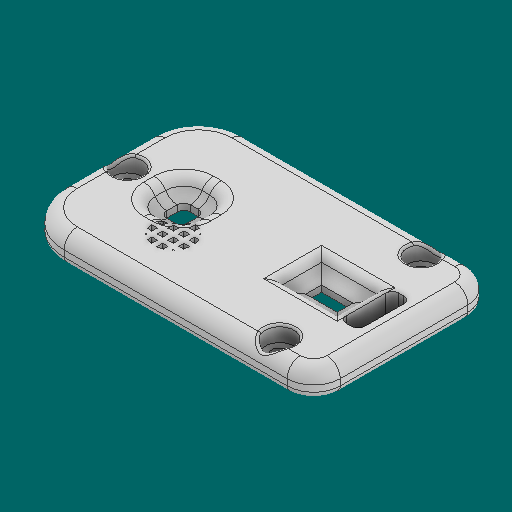
# Autodesk Inventor part: vape back
Saved by Autodesk Inventor 2025.1 (Build 291241000, 241)
## iProperties
Created: 2026-08-30
Part Number: vape back
Material: Generic
Document SubType Name: Modeling
Designer: Luke Buonanno
Density: 1 g/cm^3
Appearance: Default
Author: Luke Buonanno
Autodesk Inventor part; units mm, degrees
ref_plane "YZ Plane" through (0, 0, 0) normal (1, 0, 0) x (0, 1, 0)
ref_plane "XZ Plane" through (0, 0, 0) normal (0, 1, 0) x (-1, 0, 0)
ref_plane "XY Plane" through (0, 0, 0) normal (0, 0, 1) x (1, 0, 0)
sketch "Sketch1" plane through (0, 0, 0) normal (1, 0, 0) x (0, 1, 0)
  point P0 (0, 0)
sketch "Sketch2" plane through (0, 0, 0) normal (0, 1, 0) x (-1, 0, 0)
  point P0 (0, 0)
sketch "Sketch3" plane through (0, 0, 0) normal (0, 1, 0) x (-1, 0, 0)
  line L0 (24.5772, 9.7458) -> (-30.4138, 9.7458)
  line L1 (-30.4138, 9.7458) -> (-30.4138, -21.7502)
  line L2 (-30.4138, -21.7502) -> (24.5772, -21.7502)
  line L3 (24.5772, -21.7502) -> (24.5772, 9.7458)
  point P0 (0, 0)
  dimension "d0" = 54.991
  dimension "d1" = 31.496
  constraints: 8 end point, 2 parallel, 1 horizontal, 1 perpendicular
  measures "d0" distance of L1.end L2.end
  measures "d1" distance of L2.end L0.start
extrude "Extrusion1" add sketch "Sketch3" along normal blind 5
sketch "Sketch4" plane through (0, 5, 0) normal (0, 1, 0) x (1, 0, 0)
  line L0 (-24.5772, 21.7502) -> (-24.5772, -9.7458) projected
  line L1 (-24.5772, 6.0022) -> (-22.3166, 6.0022)
  circle A0 centre (-22.3166, 6.0022) radius 2.8
  point P0 (0, 0)
  dimension "d4" = 2.2606
  dimension "d5" = 5.6
  constraints: 2 end point, 1 centre point, 1 coincident, 1 horizontal, 1 midpoint
  measures "d4" distance of L1.start L1.end
  measures "d5" diameter of A0
sketch "Sketch5" plane through (0, 5, 0) normal (0, 1, 0) x (1, 0, 0)
  line L0 (30.4138, -9.7458) -> (30.4138, 21.7502) projected
  line L1 (30.4138, 21.7502) -> (-24.5772, 21.7502) projected
  line L2 (-24.5772, 21.7502) -> (-24.5772, -9.7458) projected
  line L3 (-24.5772, -9.7458) -> (30.4138, -9.7458) projected
  line L4 (30.4138, -11.2458) -> (-26.0772, -11.2458)
  line L5 (-26.0772, -11.2458) -> (-26.0772, 23.2502)
  line L6 (-26.0772, 23.2502) -> (30.4138, 23.2502)
  line L7 (30.4138, 23.2502) -> (30.4138, -11.2458)
  line L8 (30.4138, -11.2458) -> (-26.0772, 23.2502) construction
  line L9 (-26.0772, -11.2458) -> (30.4138, 23.2502) construction
  point P0 (0, 0)
  point P1 (2.1683, 6.0022)
  dimension "d6" = 1.5
  dimension "d7" = 1.5
  dimension "d8" = 1.5
  dimension "d9" = 0
  constraints: 12 end point, 2 midpoint, 2 parallel, 1 horizontal, 1 perpendicular
  measures "d6" distance between parallel lines of L5 L2
  measures "d7" distance between parallel lines of L6 L1
  measures "d8" distance between parallel lines of L4 L3
  measures "d9" distance between parallel lines of L0 L7
extrude "Extrusion2" add sketch "Sketch5" against normal blind 5
extrude "Extrusion3" cut sketch "Sketch4" against normal blind 3
sketch "Sketch6" plane through (-22.3166, 2, -6.0022) normal (0, 1, 0) x (1, 0, 0)
  circle A0 centre (0, 0) radius 2.8 projected
  circle A1 centre (0, 0) radius 1.5
  point P0 (22.3166, -6.0022)
  dimension "d14" = 3
  constraints: 1 centre point, 1 coincident
  measures "d14" diameter of A1
extrude "Extrusion4" cut sketch "Sketch6" against normal blind 3 contours A1
sketch "Sketch7" plane through (0, 5, 0) normal (0, 1, 0) x (1, 0, 0)
  circle A0 centre (-22.3166, 6.0022) radius 2.8 projected
  line L0 (30.4138, -11.2458) -> (30.4138, 23.2502) projected
  line L1 (30.4138, 23.2502) -> (-26.0772, 23.2502) projected
  line L2 (-26.0772, -11.2458) -> (30.4138, -11.2458) projected
  line L3 (30.4138, -9.7458) -> (-22.3166, -9.7458)
  line L4 (-22.3166, -9.7458) -> (-22.3166, 21.7502)
  line L5 (-22.3166, 21.7502) -> (30.4138, 21.7502)
  line L6 (30.4138, 21.7502) -> (30.4138, -9.7458)
  line L7 (30.4138, -9.7458) -> (-22.3166, 21.7502) construction
  line L8 (-22.3166, -9.7458) -> (30.4138, 21.7502) construction
  line L9 (30.4138, -9.7458) -> (9.8906, -9.7458)
  line L10 (20.1522, -9.7458) -> (20.1522, 21.7502)
  line L11 (20.1522, -9.7458) -> (20.1522, -7.4852)
  line L12 (20.1522, 21.7502) -> (20.1522, 19.4896)
  circle A1 centre (20.1522, -7.4852) radius 2.75
  circle A2 centre (20.1522, 19.4896) radius 2.75
  point P0 (0, 0)
  point P1 (4.0486, 6.0022)
  dimension "d17" = 1.5
  dimension "d18" = 1.5
  dimension "d19" = 0
  dimension "d20" = 10.2616
  dimension "d21" = 2.2606
  dimension "d22" = 2.2606
  dimension "d23" = 5.5
  dimension "d24" = 5.5
  dimension "d25" = 5.6
  constraints: 20 end point, 4 point on line, 3 midpoint, 2 centre point, 2 coincident, 2 parallel, 2 perpendicular, 1 horizontal
  measures "d17" distance between parallel lines of L1 L5
  measures "d18" distance between parallel lines of L2 L3
  measures "d19" distance between parallel lines of L0 L6
  measures "d20" distance of L3.start L10.start
  measures "d21" distance of L10.start L11.end
  measures "d22" distance of L10.end L12.end
  measures "d23" diameter of A1
  measures "d24" diameter of A2
  measures "d25" diameter of A0
extrude "Extrusion5" cut sketch "Sketch7" against normal blind 3 contours A2 L5 | L5 L10 A2 | L5 A2 L10 | A1 L10 L3 | L3 A1 | A1 L3 L10
sketch "Sketch8" plane through (20.1522, 2, 7.4852) normal (0, 1, 0) x (1, 0, 0)
  circle A0 centre (0, 0) radius 2.75 projected
  circle A1 centre (0, 0) radius 1.5
  circle A2 centre (0, 26.9748) radius 2.75 projected
  circle A3 centre (0, 26.9748) radius 1.5
  point P0 (-20.1522, 7.4852)
  dimension "d28" = 3
  dimension "d29" = 3
  constraints: 2 centre point, 2 coincident
  measures "d28" diameter of A1
  measures "d29" diameter of A3
extrude "Extrusion6" cut sketch "Sketch8" against normal blind 3 contours A1 | A3
sketch "Sketch9" plane through (0, 0, 0) normal (0, -1, 0) x (1, 0, 0)
  circle A0 centre (20.1522, -19.4896) radius 1.5 projected
  circle A1 centre (20.1522, 7.4852) radius 1.5 projected
  circle A2 centre (-22.3166, -6.0022) radius 1.5 projected
  line L0 (26.6532, -20.9896) -> (-22.3166, -20.9896)
  line L1 (-22.3166, -20.9896) -> (-22.3166, 8.9852)
  line L2 (-22.3166, 8.9852) -> (26.6532, 8.9852)
  line L3 (26.6532, 8.9852) -> (26.6532, -20.9896)
  line L4 (26.6532, -20.9896) -> (-22.3166, 8.9852) construction
  line L5 (-22.3166, -20.9896) -> (26.6532, 8.9852) construction
  point P0 (0, 0)
  point P1 (2.1683, -6.0022)
  point P2 (20.1522, 8.9852)
  point P3 (-22.3166, -4.5022)
  point P4 (-22.3166, -7.5022)
  point P5 (20.1522, -20.9896)
  constraints: 12 end point, 2 midpoint, 2 parallel, 1 horizontal, 1 perpendicular
extrude "Extrusion7" cut sketch "Sketch9" against normal blind 1.25 contours L0 L1 A2 L2 L3
sketch "Sketch11" plane through (0, 1.25, 0) normal (0, -1, 0) x (1, 0, 0)
  line L0 (26.6532, 8.9852) -> (26.6532, -20.9896) projected
  line L1 (26.6532, 8.9852) -> (26.6532, -20.9896) projected
  line L2 (26.6532, -20.9896) -> (26.6532, 8.9852)
  line L3 (26.6532, -6.0022) -> (24.9032, -6.0022)
  line L4 (24.4232, -11.0022) -> (25.3832, -11.0022)
  line L5 (26.6532, -9.7322) -> (26.6532, -2.2722)
  line L6 (25.3832, -1.0022) -> (24.4232, -1.0022)
  line L7 (23.1532, -2.2722) -> (23.1532, -9.7322)
  line L8 (23.1532, -11.0022) -> (26.6532, -1.0022) construction
  line L9 (26.6532, -11.0022) -> (23.1532, -1.0022) construction
  arc A0 (23.1532, -9.7322) -> (24.4232, -11.0022) centre (24.4232, -9.7322) ccw
  arc A1 (25.3832, -11.0022) -> (26.6532, -9.7322) centre (25.3832, -9.7322) ccw
  arc A2 (26.6532, -2.2722) -> (25.3832, -1.0022) centre (25.3832, -2.2722) ccw
  arc A3 (24.4232, -1.0022) -> (23.1532, -2.2722) centre (24.4232, -2.2722) ccw
  point P0 (0, 0)
  dimension "d35" = 1.75
  dimension "d36" = 3.5
  dimension "d37" = 3.5
  dimension "d38" = 10
  dimension "d39" = 1.27
  constraints: 16 end point, 9 point on line, 8 point on circle, 8 tangent, 4 centre point, 3 equal length, 3 equal radius, 3 midpoint, 2 horizontal, 1 perpendicular
  measures "d35" distance of L3.start L3.end
  measures "d36" distance of L8.end L9.end
  measures "d37" distance of L8.start L9.start
  measures "d38" distance of L9.end L8.start
  measures "d39" radius of A0
extrude "Extrusion8" cut sketch "Sketch11" against normal blind 5
sketch "Sketch12" plane through (0, 5, 0) normal (0, 1, 0) x (1, 0, 0)
  line L0 (23.1532, 9.7322) -> (23.1532, 2.2722) projected
  line L1 (23.1532, 6.0022) -> (13.1532, 6.0022)
  line L2 (23.1532, 6.0022) -> (19.1532, 6.0022)
  line L3 (19.1532, 6.0022) -> (13.1532, 6.0022)
  line L4 (19.1532, 4.5022) -> (13.1532, 4.5022)
  line L5 (13.1532, 4.5022) -> (13.1532, 7.5022)
  line L6 (13.1532, 7.5022) -> (19.1532, 7.5022)
  line L7 (19.1532, 7.5022) -> (19.1532, 4.5022)
  line L8 (19.1532, 4.5022) -> (13.1532, 7.5022) construction
  line L9 (13.1532, 4.5022) -> (19.1532, 7.5022) construction
  point P0 (0, 0)
  point P1 (16.1532, 6.0022)
  dimension "d42" = 10
  dimension "d43" = 4
  dimension "d44" = 3
  constraints: 18 end point, 4 midpoint, 2 horizontal, 2 parallel, 1 collinear, 1 perpendicular, 1 point on line
  measures "d42" distance of L1.start L1.end
  measures "d43" distance of L1.start L2.end
  measures "d44" distance of L4.end L5.end
extrude "Extrusion9" cut sketch "Sketch12" against normal blind 5
fillet "Fillet1" radius 2.54 4 edges at (-26.0772, 5, -6.0022) (2.1683, 5, 11.2458) (2.1683, 5, -23.2502) (30.4138, 5, -6.0022)
fillet "Fillet3" radius 2.54 4 edges at (13.1532, 5, -6.0022) (16.1532, 5, -7.5022) (19.1532, 5, -6.0022) (16.1532, 5, -4.5022) inverted yes
fillet "Fillet4" radius 1.905 4 edges at (10.6132, 5, -6.0022) (16.1532, 5, -10.0422) (16.1532, 5, -1.9622) (21.6932, 5, -6.0022)
fillet "Fillet5" radius 0.381 9 edges at (-20.8296, 5, -8.3747) (-20.8296, 5, -3.6297) (-25.1166, 4.4492, -6.0021) (20.1522, 4.4879, -22.2396) (22.8298, 5, -20.1164) (19.5254, 5, -16.812) (20.1522, 4.4879, 10.2352) (22.8298, 5, 8.112) (19.5254, 5, 4.8076)
fillet "Fillet6" radius 5.08 4 edges at (30.4138, 1.23, -23.2502) (29.6698, 4.2561, -22.5062) (30.4138, 1.23, 11.2458) (29.6698, 4.2561, 10.5019)
fillet "Fillet7" radius 8.89 4 edges at (-26.0772, 1.23, 11.2458) (-25.3333, 4.2561, 10.5019) (-26.0772, 1.23, -23.2502) (-25.3333, 4.2561, -22.5062)
fillet "Fillet8" radius 1.27 8 edges at (-23.4734, 0, -20.6464) (4.0733, 0, -23.2502) (28.9259, 0, -21.7623) (30.4138, 0, -6.0022) (28.9259, 0, 9.7579) (4.0733, 0, 11.2458) (-23.4734, 0, 8.642) (-26.0772, 0, -6.0022)
sketch "Sketch13" plane through (0, 1.25, 0) normal (0, -1, 0) x (1, 0, 0)
  line L0 (23.1532, -9.7322) -> (23.1532, -2.2722) projected
  line L1 (23.1532, -6.0022) -> (-9.8468, -6.0022)
  line L2 (-9.8468, -6.0022) -> (-13.8468, -6.0022)
  line L3 (-11.1168, -8.2522) -> (-12.5768, -8.2522)
  line L4 (-13.8468, -6.9822) -> (-13.8468, -5.0222)
  line L5 (-12.5768, -3.7522) -> (-11.1168, -3.7522)
  line L6 (-9.8468, -5.0222) -> (-9.8468, -6.9822)
  line L7 (-9.8468, -8.2522) -> (-13.8468, -3.7522) construction
  line L8 (-13.8468, -8.2522) -> (-9.8468, -3.7522) construction
  arc A0 (-13.8468, -6.9822) -> (-12.5768, -8.2522) centre (-12.5768, -6.9822) ccw
  arc A1 (-12.5768, -3.7522) -> (-13.8468, -5.0222) centre (-12.5768, -5.0222) ccw
  arc A2 (-9.8468, -5.0222) -> (-11.1168, -3.7522) centre (-11.1168, -5.0222) ccw
  arc A3 (-11.1168, -8.2522) -> (-9.8468, -6.9822) centre (-11.1168, -6.9822) ccw
  point P0 (0, 0)
  point P1 (-11.8468, -6.0022)
  dimension "d55" = 33
  dimension "d56" = 4
  dimension "d57" = 4.5
  dimension "d58" = 1.27
  constraints: 16 end point, 8 point on circle, 8 point on line, 8 tangent, 4 centre point, 4 midpoint, 3 equal radius, 3 horizontal, 2 parallel, 1 perpendicular
  measures "d55" distance of L1.start L1.end
  measures "d56" distance of L1.end L2.end
  measures "d57" distance of L8.start L7.end
  measures "d58" radius of A0
extrude "Extrusion10" cut sketch "Sketch13" against normal blind 5
fillet "Fillet9" radius 2.54 8 edges at (-10.2188, 5, -4.1241) (-11.8468, 5, -3.7522) (-13.4749, 5, -4.1241) (-13.8468, 5, -6.0022) (-13.4749, 5, -7.8802) (-11.8468, 5, -8.2522) (-10.2188, 5, -7.8802) (-9.8468, 5, -6.0022) inverted yes
fillet "Fillet10" radius 2.54 8 edges at (-16.3868, 5, -6.0022) (-15.2709, 5, -2.3281) (-11.8468, 5, -1.2122) (-8.4228, 5, -2.3281) (-7.3068, 5, -6.0022) (-8.4228, 5, -9.6762) (-11.8468, 5, -10.7922) (-15.2709, 5, -9.6762)
sketch "Sketch14" plane through (0, 5, 0) normal (0, 1, 0) x (1, 0, 0)
  line L0 (-11.8468, 6.0022) -> (23.1532, 6.0022)
  line L1 (23.1532, 9.7322) -> (23.1532, 2.2722) projected
  line L2 (-11.8468, 6.0022) -> (-11.8468, -0.7478)
  line L3 (-11.8468, -0.7478) -> (-6.8468, -0.7478)
  circle A0 centre (-6.8468, -0.7478) radius 3.7084
  arc A1 (-11.1168, 1.5525) -> (-7.6471, 5.0222) centre (-11.1168, 5.0222) ccw projected
  line L4 (-1.9858, -0.2393) -> (-11.7079, -0.2393)
  line L5 (-11.7079, -0.2393) -> (-11.7079, -1.2564)
  line L6 (-11.7079, -1.2564) -> (-1.9858, -1.2564)
  line L7 (-1.9858, -1.2564) -> (-1.9858, -0.2393)
  line L8 (-1.9858, -0.2393) -> (-11.7079, -1.2564) construction
  line L9 (-11.7079, -0.2393) -> (-1.9858, -1.2564) construction
  line L10 (-6.8468, -0.7478) -> (-6.8468, 2.9606)
  line L11 (-6.8468, -0.7478) -> (-6.8468, -4.4563)
  line L12 (-6.8468, -1.2564) -> (-6.8468, -2.2734)
  line L13 (-6.8468, -0.2393) -> (-6.8468, 0.7778)
  line L14 (-6.8468, -2.2734) -> (-6.8468, -3.2905)
  line L15 (-3.4667, -3.2905) -> (-10.2269, -3.2905)
  line L16 (-10.2269, -3.2905) -> (-10.2269, -2.2734)
  line L17 (-10.2269, -2.2734) -> (-3.4667, -2.2734)
  line L18 (-3.4667, -2.2734) -> (-3.4667, -3.2905)
  line L19 (-3.4667, -3.2905) -> (-10.2269, -2.2734) construction
  line L20 (-10.2269, -3.2905) -> (-3.4667, -2.2734) construction
  line L21 (-6.8468, 0.7778) -> (-6.8468, 1.7949)
  line L22 (-3.4667, 1.7949) -> (-10.2269, 1.7949)
  line L23 (-10.2269, 1.7949) -> (-10.2269, 0.7778)
  line L24 (-10.2269, 0.7778) -> (-3.4667, 0.7778)
  line L25 (-3.4667, 0.7778) -> (-3.4667, 1.7949)
  line L26 (-3.4667, 1.7949) -> (-10.2269, 0.7778) construction
  line L27 (-10.2269, 1.7949) -> (-3.4667, 0.7778) construction
  line L28 (-6.3383, 3.2402) -> (-7.3554, 3.2402)
  line L29 (-7.3554, 3.2402) -> (-7.3554, -4.7359)
  line L30 (-7.3554, -4.7359) -> (-6.3383, -4.7359)
  line L31 (-6.3383, -4.7359) -> (-6.3383, 3.2402)
  line L32 (-6.3383, 3.2402) -> (-7.3554, -4.7359) construction
  line L33 (-7.3554, 3.2402) -> (-6.3383, -4.7359) construction
  line L34 (-7.3554, -0.7478) -> (-8.3724, -0.7478)
  line L35 (-8.3724, -4.1279) -> (-9.3895, -4.1279)
  line L36 (-9.3895, -4.1279) -> (-9.3895, 2.6272)
  line L37 (-9.3895, 2.6272) -> (-8.3724, 2.6272)
  line L38 (-8.3724, 2.6272) -> (-8.3724, -4.1279)
  line L39 (-6.3383, -0.7478) -> (-5.3212, -0.7478)
  line L40 (-5.3212, -4.1279) -> (-4.3042, -4.1279)
  line L41 (-4.3042, -4.1279) -> (-4.3042, 2.6272)
  line L42 (-4.3042, 2.6272) -> (-5.3212, 2.6272)
  line L43 (-5.3212, 2.6272) -> (-5.3212, -4.1279)
  point P0 (0, 0)
  point P1 (-6.8468, -2.782)
  point P2 (-6.8468, 1.2863)
  point P3 (-9.3895, -3.4473)
  point P4 (-9.3895, -3.2905)
  point P5 (-9.5463, -3.2905)
  point P6 (-9.3895, 1.7949)
  point P7 (-9.3895, 1.9517)
  point P8 (-9.5463, 1.7949)
  point P9 (-4.3042, -3.2905)
  point P10 (-4.3042, -3.4473)
  point P11 (-4.1473, -3.2905)
  point P12 (-4.3042, 1.9517)
  point P13 (-4.3042, 1.7949)
  point P14 (-4.1473, 1.7949)
  point P15 (-5.3212, 1.7949)
  point P16 (-5.31, 2.6272)
  point P17 (-6.3383, 2.9256)
  point P18 (-6.3383, 1.7949)
  point P19 (-5.3212, -0.2393)
  point P20 (-5.3212, 0.7778)
  point P21 (-6.3383, 0.7778)
  point P22 (-6.3383, -0.2393)
  point P23 (-4.3042, 0.7778)
  point P24 (-4.3042, -0.2393)
  point P25 (-3.1734, -0.2393)
  point P26 (-4.3042, -1.2564)
  point P27 (-4.3042, -2.2734)
  point P28 (-3.1734, -1.2564)
  point P29 (-5.3212, -3.2905)
  point P30 (-6.3383, -3.2905)
  point P31 (-6.3383, -4.4212)
  point P32 (-5.3212, -2.2734)
  point P33 (-5.3212, -1.2564)
  point P34 (-6.3383, -1.2564)
  point P35 (-6.3383, -2.2734)
  point P36 (-8.3724, -1.2564)
  point P37 (-8.3724, -2.2734)
  point P38 (-7.3554, -2.2734)
  point P39 (-7.3554, -1.2564)
  point P40 (-8.3724, -3.2905)
  point P41 (-7.3554, -4.4212)
  point P42 (-7.3554, -3.2905)
  point P43 (-9.3895, -2.2734)
  point P44 (-9.3895, -1.2564)
  point P45 (-10.5202, -1.2564)
  point P46 (-9.3895, -0.2393)
  point P47 (-9.3895, 0.7778)
  point P48 (-10.5202, -0.2393)
  point P49 (-8.3724, -0.2393)
  point P50 (-7.3554, -0.2393)
  point P51 (-7.3554, 0.7778)
  point P52 (-8.3724, 0.7778)
  point P53 (-8.3724, 1.7949)
  point P54 (-7.3554, 1.7949)
  point P55 (-7.3554, 2.9256)
  point P56 (-8.3837, 2.6272)
  dimension "d63" = 6.75
  dimension "d64" = 5
  dimension "d65" = 1.0171
  dimension "d66" = 1.0171
  dimension "d67" = 1.0171
  dimension "d68" = 1.0171
  dimension "d69" = 1.0171
  dimension "d70" = 1.0171
  dimension "d71" = 1.0171
  dimension "d72" = 1.0171
  dimension "d73" = 1.0171
  dimension "d74" = 1.0171
  constraints: 86 end point, 15 midpoint, 12 parallel, 8 perpendicular, 8 point on line, 6 horizontal, 2 vertical, 1 coincident, 9 other
  measures "d63" distance of L0.start L2.end
  measures "d64" distance of L2.end L3.end
  measures "d65" distance of L4.end L5.end
  measures "d66" distance of L12.start L12.end
  measures "d67" distance of L13.start L13.end
  measures "d68" distance of L14.end L12.end
  measures "d69" distance of L13.end L21.end
  measures "d70" distance of L28.start L28.end
  measures "d71" distance of L34.end L34.start
  measures "d72" distance of L36.end L37.end
  measures "d73" distance of L39.start L39.end
  measures "d74" distance of L41.end L42.end
extrude "Extrusion11" cut sketch "Sketch14" against normal blind 10 contours L4 L38 L24 L29 | L29 L17 L38 L6 | L36 L17 A0 L6 | L4 A0 L24 L36 | L31 L24 L43 L4 | L6 L43 L17 L31 | L22 L38 L37 A0 L29 | L29 A0 L38 L15 | L36 A0 L15 | L22 A0 L36 | L41 L24 A0 L4 | L31 A0 L42 L43 L22 | L6 A0 L17 L41 | L15 L43 A0 L31 | L41 A0 L22 | L15 A0 L41
body "Solid1"
